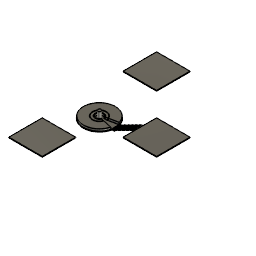
GameJam Skull Room (Autodesk Fusion 360 design; units mm, degrees)
Autodesk Fusion 360 part; units mm, degrees
note: some values were not read from the file. Chosen so that the rebuilt part matches the saved one: a side.
sketch "Sketch1" plane through (0, 0, 0) normal (0, 0, 1) x (1, 0, 0)
  circle A0 centre (0, 0) radius 50
  circle A1 centre (0, 0) radius 62
  circle A2 centre (0, 0) radius 102
  circle A3 centre (0, 0) radius 242
  circle A4 centre (172, 0) radius 50
  line L0 (0, 0) -> (242, 0) construction
  line L1 (102, 0) -> (242, 0) construction
  circle A5 centre (121.6224, 121.6224) radius 50
  circle A6 centre (0, 172) radius 50
  circle A7 centre (-121.6224, 121.6224) radius 50
  circle A8 centre (-172, 0) radius 50
  circle A9 centre (-121.6224, -121.6224) radius 50
  circle A10 centre (0, -172) radius 50
  circle A11 centre (121.6224, -121.6224) radius 50
  line L2 (62, 0) -> (102, 0) construction
  circle A12 centre (82, 0) radius 10
  circle A13 centre (71.0141, 41) radius 10
  circle A14 centre (41, 71.0141) radius 10
  circle A15 centre (0, 82) radius 10
  circle A16 centre (-41, 71.0141) radius 10
  circle A17 centre (-71.0141, 41) radius 10
  circle A18 centre (-82, 0) radius 10
  circle A19 centre (-71.0141, -41) radius 10
  circle A20 centre (-41, -71.0141) radius 10
  circle A21 centre (0, -82) radius 10
  circle A22 centre (41, -71.0141) radius 10
  circle A23 centre (71.0141, -41) radius 10
  line L3 (50, 0) -> (62, 0) construction
  circle A24 centre (56, 0) radius 2
  circle A25 centre (53.2592, 17.305) radius 2
  circle A26 centre (45.305, 32.916) radius 2
  circle A27 centre (32.916, 45.305) radius 2
  circle A28 centre (17.305, 53.2592) radius 2
  circle A29 centre (0, 56) radius 2
  circle A30 centre (-17.305, 53.2592) radius 2
  circle A31 centre (-32.916, 45.305) radius 2
  circle A32 centre (-45.305, 32.916) radius 2
  circle A33 centre (-53.2592, 17.305) radius 2
  circle A34 centre (-56, 0) radius 2
  circle A35 centre (-53.2592, -17.305) radius 2
  circle A36 centre (-45.305, -32.916) radius 2
  circle A37 centre (-32.916, -45.305) radius 2
  circle A38 centre (-17.305, -53.2592) radius 2
  circle A39 centre (0, -56) radius 2
  circle A40 centre (17.305, -53.2592) radius 2
  circle A41 centre (32.916, -45.305) radius 2
  circle A42 centre (45.305, -32.916) radius 2
  circle A43 centre (53.2592, -17.305) radius 2
  line L4 (44.6514, 22.5) -> (233.7386, 62.6917)
  line L5 (44.6514, -22.5) -> (233.7386, -62.6917)
  line L6 (44.6514, 22.5) -> (44.6514, -22.5) construction
  circle A44 centre (0, 0) radius 25
  line L7 (250, 1102) -> (-250, 1102)
  line L8 (-250, 1102) -> (-250, 602)
  line L9 (-250, 602) -> (250, 602)
  line L10 (250, 602) -> (250, 1102)
  line L11 (250, 1102) -> (-250, 602) construction
  line L12 (-250, 1102) -> (250, 602) construction
  line L13 (250, -602) -> (-250, -602)
  line L14 (-250, -602) -> (-250, -1102)
  line L15 (-250, -1102) -> (250, -1102)
  line L16 (250, -1102) -> (250, -602)
  line L17 (250, -602) -> (-250, -1102) construction
  line L18 (-250, -602) -> (250, -1102) construction
  line L19 (1102, 250) -> (602, 250)
  line L20 (602, 250) -> (602, -250)
  line L21 (602, -250) -> (1102, -250)
  line L22 (1102, -250) -> (1102, 250)
  line L23 (1102, 250) -> (602, -250) construction
  line L24 (602, 250) -> (1102, -250) construction
  line L25 (0, 0) -> (0, 852) construction
  line L26 (0, 0) -> (0, -852) construction
  line L27 (0, 0) -> (852, 0) construction
  line L28 (236.7784, 50) -> (272, 50)
  line L29 (272, 50) -> (272, -50)
  line L30 (272, -50) -> (236.7784, -50)
  point P0 (0, 852)
  point P1 (0, -852)
  point P2 (852, 0)
  point P3 (242, 0)
  dimension "d1" = 100
  dimension "d2" = 40
  dimension "d3" = 140
  dimension "d4" = 12
  dimension "d6" = 100
  dimension "d8" = 360
  dimension "d9" = 20
  dimension "d11" = 360
  dimension "d12" = 4
  dimension "d14" = 360
  dimension "d15" = 12
  dimension "d16" = 45
  dimension "d28" = 50
  dimension "d31" = 500
  dimension "d32" = 360
  dimension "d44" = 100
  dimension "d45" = 30
  constraint coincident A0.centre A1.centre
  constraint concentric A0 A1
  constraint concentric A0 A2
  constraint concentric A0 A3
  constraint coincident A3 P3
  constraint horizontal L0
  constraint coincident A2 L1.start
  constraint coincident L0 L1.start
  constraint midpoint A4.centre L1
  constraint coincident A1 L2.start
  constraint coincident L0 L2.start
  constraint midpoint L2 A12.centre
  constraint coincident A0 L3.start
  constraint coincident L0 L3.start
  constraint midpoint L3 A24.centre
  constraint coincident A0 L4.start
  constraint coincident A3 L4.end
  constraint coincident A0 L5.start
  constraint coincident A3 L5.end
  constraint symmetric L0 L4.end L5.end
  constraint symmetric L1 L4.start L5.start
  constraint concentric A2 A44
  constraint horizontal L7
  constraint perpendicular L7 L8
  constraint parallel L7 L9
  constraint parallel L8 L10
  constraint coincident L11 P0
  constraint coincident L12 P0
  constraint horizontal L13
  constraint perpendicular L13 L14
  constraint parallel L13 L15
  constraint parallel L14 L16
  constraint coincident L17 P1
  constraint coincident L18 P1
  constraint horizontal L19
  constraint perpendicular L19 L20
  constraint parallel L19 L21
  constraint parallel L20 L22
  constraint coincident L23 P2
  constraint coincident L24 P2
  constraint equal L7 L8
  constraint equal L10 L19
  constraint equal L20 L21
  constraint equal L14 L15
  constraint equal L13 L20
  constraint coincident P0 L25.end
  constraint vertical L25
  constraint coincident P1 L26.end
  constraint vertical L26
  constraint coincident P2 L27.end
  constraint horizontal L27
  constraint equal L25 L27
  constraint equal L26 L27
  constraint coincident P3 L0.end
  constraint coincident A3 L28.start
  constraint horizontal L28
  constraint coincident A3 L30.end
  constraint parallel L28 L30
  constraint equal L28 L30
  constraint vertical L29
  measures "d1" diameter of A0
  measures "d2" distance of A1 A2
  measures "d3" distance of A2 A3
  measures "d4" distance of A0 A1
  measures "d6" diameter of A4
  measures "d9" diameter of A12
  measures "d12" diameter of A24
  measures "d15" angle of L0 L4
  measures "d16" distance of L4.start L5.start
  measures "d28" diameter of A44
  measures "d31" distance of L19.start L21.end
  measures "d32" distance of L20 P3
  measures "d44" distance of L28.end L29.end
  measures "d45" distance of P3 L29
extrude "Extrude1" add sketch "Sketch1" against normal blind 10 contours A0 | A0 A1 L4 L5 | A0 A1 L4 L5 | A1 A2 L4 L5 | A1 A2 L4 L5 | A2 A4 L4 L5 | A2 A3 A4 L4 L5 | A4 L4 L5 | A4 L4 | A4 L5 | A3 A4 L4 L5 | A5 | A6 | A7 | A8 | A9 | A10 | A11 | A12 | A13 | A14 | A15 | A16 | A17 | A18 | A19 | A20 | A21 | A22 | A23 | A24 | A25 | A26 | A27 | A28 | A29 | A30 | A31 | A32 | A33 | A34 | A35 | A36 | A37 | A38 | A39 | A40 | A41 | A42 | A43 | A44 makes body 1
extrude "Extrude2" add sketch "Sketch1" along normal blind 30 separate body contours A2 A3 A4 L4 L5 | A4 L4 | A4 L5 | A5 | A6 | A7 | A8 | A9 | A10 | A11 makes body 2
extrude "Extrude3" add sketch "Sketch1" along normal blind 30 separate body contours A1 A2 L4 L5 | A13 | A14 | A15 | A16 | A17 | A18 | A19 | A20 | A21 | A22 | A23 picked at (63.5305, -63.3152) makes body 3
extrude "Extrude4" add sketch "Sketch1" along normal blind 30 separate body contours A0 A1 L4 L5 | A26 | A27 | A28 | A29 | A30 | A31 | A32 | A33 | A34 | A35 | A36 | A37 | A38 | A39 | A40 | A41 | A42 picked at (49.2378, 26.2586) makes body 4
extrude "Extrude5" cut sketch "Sketch1" along normal blind 30 thin wall 5 centred open curves A2 A1 A0 A3 bodies 2 3 4
extrude "Extrude6" add sketch "Sketch1" along normal blind 100 separate body contours A44 makes body 5
extrude "Extrude7" add sketch "Sketch1" against normal blind 10 from surface at 180 separate body contours L7 L8 L9 L10 | L13 L14 L15 L16 | L19 L20 L21 L22 makes body 6 at (-83.3333, 768.6667, 180) makes body 7 at (768.6667, 83.3333, 180) makes body 8 at (-83.3333, -935.3333, 180)
sketch "Sketch2" plane through (0, 0, 0) normal (0, 1, 0) x (1, 0, 0)
  line L0 (602, -180) -> (602, -170)
  line L1 (-242, 0) -> (242, 0)
  line L2 (242, 10) -> (-242, 10)
  line L3 (242, 0) -> (242, -10)
  line L4 (242, -10) -> (262, -10)
  line L5 (262, -10) -> (262, -20)
  line L6 (262, -20) -> (282, -20)
  line L7 (282, -20) -> (282, -30)
  line L8 (282, -30) -> (302, -30)
  line L9 (302, -30) -> (302, -40)
  line L10 (302, -40) -> (322, -40)
  line L11 (322, -40) -> (322, -50)
  line L12 (322, -50) -> (342, -50)
  line L13 (342, -50) -> (342, -60)
  line L14 (342, -60) -> (362, -60)
  line L15 (362, -60) -> (362, -70)
  line L16 (362, -70) -> (382, -70)
  line L17 (382, -70) -> (382, -80)
  line L18 (382, -80) -> (402, -80)
  line L19 (442, -100) -> (442, -110)
  line L20 (502, -130) -> (502, -140)
  line L21 (542, -160) -> (562, -160)
  line L22 (462, -120) -> (482, -120)
  line L23 (422, -90) -> (422, -100)
  line L24 (422, -100) -> (442, -100)
  line L25 (542, -150) -> (542, -160)
  line L26 (442, -110) -> (462, -110)
  line L27 (482, -130) -> (502, -130)
  line L28 (522, -140) -> (522, -150)
  line L29 (402, -80) -> (402, -90)
  line L30 (502, -140) -> (522, -140)
  line L31 (522, -150) -> (542, -150)
  line L32 (482, -120) -> (482, -130)
  line L33 (402, -90) -> (422, -90)
  line L34 (462, -110) -> (462, -120)
  line L35 (562, -160) -> (562, -170)
  line L36 (562, -170) -> (582, -170)
  line L37 (582, -170) -> (582, -180)
  line L38 (582, -180) -> (602, -180)
  point P0 (402, -80)
  dimension "d36" = 10
  dimension "d37" = 20
  constraint coincident L1.end L3.start
  constraint perpendicular L1 L3
  constraint perpendicular L3 L4
  constraint perpendicular L4 L5
  constraint perpendicular L5 L6
  constraint perpendicular L6 L7
  constraint perpendicular L7 L8
  constraint perpendicular L6 L9
  constraint perpendicular L9 L10
  constraint perpendicular L6 L11
  constraint perpendicular L11 L12
  constraint perpendicular L12 L13
  constraint perpendicular L13 L14
  constraint perpendicular L14 L15
  constraint perpendicular L15 L16
  constraint equal L4 L6
  constraint equal L6 L8
  constraint equal L8 L10
  constraint equal L10 L12
  constraint equal L12 L14
  constraint equal L14 L16
  constraint equal L3 L5
  constraint equal L5 L7
  constraint equal L7 L9
  constraint equal L9 L11
  constraint equal L11 L13
  constraint equal L13 L15
  constraint perpendicular L16 L17
  constraint perpendicular L17 L18
  constraint equal L15 L17
  constraint equal L16 L18
  constraint coincident P0 L18.end
  constraint perpendicular L29 L33
  constraint perpendicular L23 L33
  constraint perpendicular L23 L24
  constraint perpendicular L19 L24
  constraint perpendicular L19 L26
  constraint perpendicular L24 L34
  constraint perpendicular L22 L34
  constraint perpendicular L24 L32
  constraint perpendicular L27 L32
  constraint perpendicular L20 L27
  constraint perpendicular L20 L30
  constraint perpendicular L28 L30
  constraint perpendicular L28 L31
  constraint equal L24 L33
  constraint equal L24 L26
  constraint equal L22 L26
  constraint equal L22 L27
  constraint equal L27 L30
  constraint equal L30 L31
  constraint equal L23 L29
  constraint equal L19 L23
  constraint equal L19 L34
  constraint equal L32 L34
  constraint equal L20 L32
  constraint equal L20 L28
  constraint perpendicular L25 L31
  constraint perpendicular L21 L25
  constraint equal L25 L28
  constraint equal L21 L31
  constraint horizontal L33
  constraint perpendicular L21 L35
  constraint perpendicular L35 L36
  constraint perpendicular L36 L37
  constraint coincident L0.start L38.end
  constraint perpendicular L37 L38
  constraint equal L35 L37
  constraint equal L36 L38
  constraint equal L17 L29
  constraint equal L18 L33
  measures "d36" distance of L1.end L3.end
  measures "d37" distance of L3.end L4.end
extrude "Extrude8" add sketch "Sketch2" along normal mid plane 100 thin wall 10 on the left separate body open curves L3 L4 L5 L6 L7 L8 L9 L10 L11 L12 L13 L14 L15 L16 L17 L18 L29 L33 L23 L24 L19 L26 L34 L22 L32 L27 L20 L30 L28 L31 L25 L21 L35 L36 L37 L38 makes body 9
extrude "Extrude9" add sketch "Sketch1" against normal blind 10 contours A3 L28 L29 L30 bodies 1
equation "scale = 5"
equation "d12 = ( 20 / 5 ) * 1 mm"
